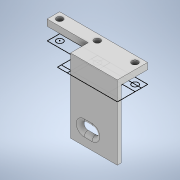
# Autodesk Inventor part: enclosure mounter
Saved by Autodesk Inventor 2022 (Build 260153000, 153)
## iProperties
Created: 2022-04-12
Part Number: enclosure mounter
Material: Generic
Document SubType Name: Modeling
Designer: a-dubs
Density: 1 g/cm^3
Appearance: Default
Author: a-dubs
Autodesk Inventor part; units mm, degrees
ref_plane "YZ Plane" through (0, 0, 0) normal (1, 0, 0) x (0, 1, 0)
ref_plane "XZ Plane" through (0, 0, 0) normal (0, 1, 0) x (-1, 0, 0)
ref_plane "XY Plane" through (0, 0, 0) normal (0, 0, 1) x (1, 0, 0)
sketch "Sketch1" plane through (0, 0, 0) normal (0, 1, 0) x (-1, 0, 0)
  line L0 (0, 0) -> (-19.17, 0)
  circle A0 centre (0, 0) radius 1.6
  circle A1 centre (-19.17, 0) radius 1.6
  line L1 (-19.17, 0) -> (-22.37, 0)
  line L2 (0, 0) -> (3.2, 0)
  line L3 (-22.37, 0) -> (-22.37, 3.2)
  line L4 (3.2, 0) -> (3.2, -3.2)
  line L5 (3.2, -3.2) -> (-22.37, -3.2)
  line L6 (-22.37, -3.2) -> (-22.37, 3.2)
  line L7 (-22.37, 3.2) -> (3.2, 3.2)
  line L8 (3.2, 3.2) -> (3.2, -3.2)
  line L9 (3.2, 3.2) -> (3.2, 10.2)
  line L10 (3.2, 10.2) -> (3.2, 12.2)
  line L11 (3.2, 12.2) -> (-22.37, 12.2)
  line L12 (-22.37, 12.2) -> (-22.37, 10.2)
  line L13 (-22.37, 10.2) -> (3.2, 10.2)
  line L14 (-22.37, 3.2) -> (-22.37, 10.2)
  line L15 (-9.585, 12.2) -> (1.415, 12.2)
  line L16 (-9.585, 12.2) -> (-15.985, 12.2)
  line L17 (-15.985, 12.2) -> (-15.985, 10.2)
  line L18 (1.415, 12.2) -> (1.415, 10.2)
  line L19 (0, 0) -> (0, -3.2)
  circle A2 centre (19.17, 0) radius 1.6
  line L20 (22.37, 0) -> (22.37, 3.2)
  line L21 (-3.2, 0) -> (-3.2, -3.2)
  line L22 (-3.2, -3.2) -> (22.37, -3.2)
  line L23 (22.37, -3.2) -> (22.37, 3.2)
  line L24 (22.37, 3.2) -> (-3.2, 3.2)
  line L25 (-3.2, 3.2) -> (-3.2, -3.2)
  line L26 (3.2, 10.2) -> (8.2, 10.2)
  line L27 (8.2, 10.2) -> (8.2, 3.2)
  line L28 (8.2, 10.2) -> (8.2, 12.2)
  line L29 (8.2, 12.2) -> (3.2, 12.2)
  line L30 (1.415, 10.2) -> (1.415, 3.2)
  line L31 (-15.985, 10.2) -> (-15.985, 3.2)
  point P0 (3.2, 3.2)
  point P1 (3.2, 3.2)
  point P2 (1.415, 3.2)
  dimension "d0" = 19.17
  dimension "d1" = 3.2
  dimension "d2" = 3.2
  dimension "d3" = 3.2
  dimension "d4" = 3.2
  dimension "d5" = 3.2
  dimension "d6" = 3.2
  dimension "d7" = 7
  dimension "d8" = 2
  dimension "d21" = 11
  dimension "d22" = 6.4
  dimension "d30" = 5
  constraints: 64 end point, 11 perpendicular, 10 point on line, 7 symmetric about line, 5 horizontal, 3 centre point, 3 vertical, 2 coincident, 2 parallel, 1 collinear, 1 midpoint, 1 other
  measures "d0" distance of L0.start L0.end
  measures "d1" diameter of A0
  measures "d2" diameter of A1
  measures "d3" distance of L1.start L1.end
  measures "d4" distance of L2.start L2.end
  measures "d5" distance of L1.end L3.end
  measures "d6" distance of L2.end L4.end
  measures "d7" distance of L7.end L9.end
  measures "d8" distance of L9.end L10.end
  measures "d21" distance of L15.start L15.end
  measures "d22" distance of L15.start L16.end
  measures "d30" distance of L9.end L26.end
extrude "Extrusion1" add sketch "Sketch1" along normal blind 6.4 contours L17 L11 L18 L13 | L13 L12 L11 L17
extrude "Extrusion2" add sketch "Sketch1" along normal blind 3.2 from surface at 6.4 contours L21 L5 L6 L1 A1 L0 | L25 L7 L8 L2 A0 L0 | L0 A0 L19 L5 L21 | L0 A1 L1 L3 L7 L25 | L7 L31 L13 L30 | L2 L4 L5 L19 A0 | L7 L14 L13 L31 | L8 L24 L20 L23 L22 L4 | L17 L11 L18 L13 | L13 L12 L11 L17
extrude "Extrusion3" add sketch "Sketch1" against normal blind 28 contours L17 L11 L18 L13 | L13 L12 L11 L17
sketch "Sketch2" plane through (-3.2, 9.6, 12.2) normal (0, 0, 1) x (1, 0, 0)
  line L0 (0, 0) -> (0, -9.6)
  line L1 (0, -9.6) -> (0, -29.6)
  line L2 (-3.2, -29.6) -> (21.33, -29.6)
  line L3 (9.065, -30.1) -> (5.865, -30.1)
  line L4 (9.065, -29.6) -> (12.265, -29.6)
  line L5 (0, -3.2) -> (0, 0) projected
  line L6 (0, 0) -> (0, -9.6)
  arc A0 (8.665, -27.6) -> (8.665, -31.6) centre (8.665, -29.6) ccw
  line L7 (8.665, -27.6) -> (12.665, -27.6)
  line L8 (12.665, -31.6) -> (8.665, -31.6)
  arc A1 (12.665, -31.6) -> (12.665, -27.6) centre (12.665, -29.6) ccw
  point P0 (3.2, -9.6)
  point P1 (0, -30.1)
  dimension "d16" = 20
  dimension "d18" = 3.2
  dimension "d23" = 9.6
  constraints: 16 end point, 4 point on circle, 3 point on line, 2 centre point, 2 tangent, 1 midpoint, 1 perpendicular
  measures "d16" distance of L1.end L0.end
  measures "d18" distance of L4.start L4.end
  measures "d23" distance of L0.start L6.end
extrude "Extrusion4" cut sketch "Sketch2" against normal through all
fillet "Fillet1" radius 2 4 edges at (11.465, -20, 12.2) (7.465, -22, 12.2) (3.465, -20, 12.2) (7.465, -18, 12.2)
body "Solid1"
